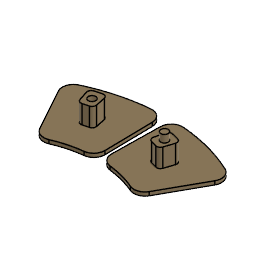
Brodie Coil (Autodesk Fusion 360 design; units mm, degrees)
Autodesk Fusion 360 part; units mm, degrees
sketch "Sketch1" plane through (0, 0, 0) normal (0, 0, 1) x (1, 0, 0)
  line L0 (0.5209, 29.8451) -> (0.7486, 42.8887)
  line L1 (14.4714, 26.1071) -> (20.796, 37.517)
  arc A0 (19.44, 41.6904) -> (4.0097, 45.8249) centre (0, 0) ccw
  arc A1 (10.6628, 24.8053) -> (3.1684, 26.8134) centre (0, 0) ccw
  arc A2 (0.5209, 29.8451) -> (3.1684, 26.8134) centre (3.5205, 29.7927) ccw
  arc A3 (20.796, 37.517) -> (19.44, 41.6904) centre (18.1722, 38.9714) ccw
  arc A4 (10.6628, 24.8053) -> (14.4714, 26.1071) centre (11.8475, 27.5615) ccw
  arc A5 (4.0097, 45.8249) -> (0.7486, 42.8887) centre (3.7482, 42.8363) ccw
  dimension "d9" = 3
  constraint concentric A0 A1
  constraint tangent A1 A2
  constraint tangent L0 A2
  constraint tangent L1 A3
  constraint tangent A0 A3
  constraint equal A2 A3
  constraint tangent L1 A4
  constraint tangent A1 A4
  constraint equal A2 A4
  constraint tangent L0 A5
  constraint tangent A0 A5
  constraint equal A2 A5
  measures "d9" radius of A2
extrude "Extrude1" add sketch "Sketch1" along normal blind 1 makes body 1
sketch "Sketch2" plane through (0, 0, 1) normal (0, 0, 1) x (-1, 0, 0)
  arc A0 (-10.6628, -24.8053) -> (-14.4714, -26.1071) centre (-11.8475, -27.5615) ccw
  line L0 (-14.4714, -26.1071) -> (-20.796, -37.517)
  arc A1 (-20.796, -37.517) -> (-19.44, -41.6904) centre (-18.1722, -38.9714) ccw
  arc A2 (-19.44, -41.6904) -> (-4.0097, -45.8249) centre (0, 0) ccw
  arc A3 (-4.0097, -45.8249) -> (-0.7486, -42.8887) centre (-3.7482, -42.8363) ccw
  line L1 (-0.7486, -42.8887) -> (-0.5209, -29.8451)
  arc A4 (-0.5209, -29.8451) -> (-3.1684, -26.8134) centre (-3.5205, -29.7927) ccw
  arc A5 (-10.6628, -24.8053) -> (-3.1684, -26.8134) centre (0, 0) ccw
  line L2 (0, 0) -> (46, 0) construction
  line L3 (0, 0) -> (46, 0) construction
  line L4 (0, 0) -> (46, 0) construction
  line L5 (-7.2999, -34.3435) -> (-7.8719, -37.0344)
  line L6 (-10.8498, -33.3923) -> (-11.6999, -36.0087)
  arc A6 (-9.617, -32.7419) -> (-8.0424, -33.1638) centre (0, 0) ccw
  arc A7 (-11.0327, -37.2766) -> (-9.0837, -37.7988) centre (0, 0) ccw
  arc A8 (-9.0837, -37.7988) -> (-7.8719, -37.0344) centre (-8.8501, -36.8265) ccw
  arc A9 (-9.617, -32.7419) -> (-10.8498, -33.3923) centre (-9.8988, -33.7013) ccw
  arc A10 (-7.2999, -34.3435) -> (-8.0424, -33.1638) centre (-8.2781, -34.1356) ccw
  arc A11 (-11.6999, -36.0087) -> (-11.0327, -37.2766) centre (-10.7489, -36.3177) ccw
  dimension "d25" = 1
  constraint horizontal L2
  constraint horizontal L3
  constraint horizontal L4
  constraint tangent A7 A8
  constraint tangent L5 A8
  constraint tangent L6 A9
  constraint tangent A6 A9
  constraint equal A8 A9
  constraint tangent L5 A10
  constraint tangent A6 A10
  constraint equal A8 A10
  constraint tangent A7 A11
  constraint tangent L6 A11
  constraint equal A8 A11
  measures "d25" radius of A8
extrude "Extrude2" add sketch "Sketch2" along normal blind 5 contours L5 L6 A6 A7 A8 A9 A10 A11 bodies 1
sketch "Sketch3" plane through (0, 0, 6) normal (0, 0, 1) x (-1, 0, 0)
  arc A0 (-9.617, -32.7419) -> (-10.8498, -33.3923) centre (-9.8988, -33.7013) ccw
  line L0 (-10.8498, -33.3923) -> (-11.6999, -36.0087)
  arc A1 (-11.6999, -36.0087) -> (-11.0327, -37.2766) centre (-10.7489, -36.3177) ccw
  arc A2 (-11.0327, -37.2766) -> (-9.0837, -37.7988) centre (0, 0) ccw
  arc A3 (-9.0837, -37.7988) -> (-7.8719, -37.0344) centre (-8.8501, -36.8265) ccw
  line L1 (-7.8719, -37.0344) -> (-7.2999, -34.3435)
  arc A4 (-7.2999, -34.3435) -> (-8.0424, -33.1638) centre (-8.2781, -34.1356) ccw
  arc A5 (-9.617, -32.7419) -> (-8.0424, -33.1638) centre (0, 0) ccw
  circle A6 centre (-9.4469, -35.2563) radius 1
  dimension "d29" = 36.5
  dimension "d30" = 2
  measures "d29" distance of A2.centre A6.centre
  measures "d30" diameter of A6
extrude "Extrude3" add sketch "Sketch3" along normal blind 2 contours A6 bodies 1
copy_body "CopyPasteBodies1" bodies 1 makes body 2
move_body "Move1" bodies 2 to x (1, 0, 0) y (0, 1, 0) z (0, 0, 1) at (-22, 0, 0)
extrude "Extrude4" cut 1 faces at (-12.8085, 35.6309, 8) along direction (0, 0, -1) blind 4 on bodies 2 bodies 2
move_body "Move2" bodies 2 to x (0.866025, 0.5, 0) y (-0.5, 0.866025, 0) z (0, 0, 1) at (18.4253, 10.9073, 0)
